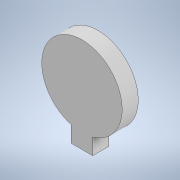
# Autodesk Inventor part: try
Saved by Autodesk Inventor 2021 (Build 250183000, 183)
## iProperties
Created: 2023-03-20
Part Number: try
Material: Generic
Document SubType Name: Modeling
Designer: mahmo
Density: 1 g/cm^3
Appearance: Default
Author: mahmo
Autodesk Inventor part; units mm, degrees
ref_plane "YZ Plane" through (0, 0, 0) normal (1, 0, 0) x (0, 1, 0)
ref_plane "XZ Plane" through (0, 0, 0) normal (0, 1, 0) x (-1, 0, 0)
ref_plane "XY Plane" through (0, 0, 0) normal (0, 0, 1) x (1, 0, 0)
sketch "Sketch1" plane through (0, 0, 0) normal (0, 0, 1) x (1, 0, 0)
  circle A0 centre (0, 0) radius 7.5
  line L0 (2, -2.25) -> (2, -10.25)
  line L1 (2, -10.25) -> (-2, -10.25)
  line L2 (-2, -10.25) -> (-2, -2.25)
  point P0 (0, 0)
  point P1 (0, 0)
  point P2 (-2, -7.2284)
  point P3 (2, -7.2284)
  constraints: 6 end point, 1 centre point
extrude "Extrusion1" add sketch "Sketch1" along normal blind 3
body "Solid1"
